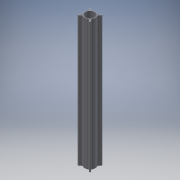
# Autodesk Inventor part: X95_1000mm
Saved by Autodesk Inventor 2016 (Build 200138000, 138)
## iProperties
Created: 2012-04-18
Part Number: X95_1000mm
Document SubType Name: Modeling
Designer: Fabian
Density: 1 g/cm^3
Material: Generic
Appearance: Default
Author: Fabian
Autodesk Inventor part; units mm, degrees
ref_plane "YZ Plane" through (0, 0, 0) normal (1, 0, 0) x (0, 1, 0)
ref_plane "XZ Plane" through (0, 0, 0) normal (0, 1, 0) x (-1, 0, 0)
ref_plane "XY Plane" through (0, 0, 0) normal (0, 0, 1) x (1, 0, 0)
sketch "Sketch1" plane through (0, 0, 0) normal (0, 0, 1) x (1, 0, 0)
  arc A0 (11.6951, -1.7956) -> (0, 0) centre (4.624, -8.8667) ccw
  line L0 (11.6951, -1.7956) -> (21.2005, -11.301)
  arc A1 (21.2005, -11.301) -> (22.9683, -12.0332) centre (22.9683, -9.5332) ccw
  line L1 (22.9683, -12.0332) -> (26.5038, -12.0332)
  arc A2 (26.5038, -12.0332) -> (29.0038, -9.5332) centre (26.5038, -9.5332) ccw
  line L2 (29.0038, -9.5332) -> (29.0038, -5.9977)
  arc A3 (29.0038, -5.9977) -> (28.2716, -4.2299) centre (26.5038, -5.9977) ccw
  line L3 (28.2716, -4.2299) -> (18.7662, 5.2754)
  arc A4 (16.9706, 16.9706) -> (18.7662, 5.2754) centre (25.8373, 12.3465) ccw
  arc A5 (16.9706, 16.9706) -> (16.9706, 53.963) centre (-18.4962, 35.4668) ccw
  arc A6 (18.7662, 65.6581) -> (16.9706, 53.963) centre (25.8373, 58.587) ccw
  line L4 (18.7662, 65.6581) -> (28.2716, 75.1635)
  arc A7 (28.2716, 75.1635) -> (29.0038, 76.9312) centre (26.5038, 76.9312) ccw
  line L5 (29.0038, 76.9312) -> (29.0038, 80.4668)
  arc A8 (29.0038, 80.4668) -> (26.5038, 82.9668) centre (26.5038, 80.4668) ccw
  line L6 (26.5038, 82.9668) -> (22.9683, 82.9668)
  arc A9 (22.9683, 82.9668) -> (21.2005, 82.2345) centre (22.9683, 80.4668) ccw
  line L7 (21.2005, 82.2345) -> (11.6951, 72.7291)
  arc A10 (0, 70.9335) -> (11.6951, 72.7291) centre (4.624, 79.8002) ccw
  arc A11 (0, 70.9335) -> (-36.9924, 70.9335) centre (-18.4962, 35.4668) ccw
  arc A12 (-48.6875, 72.7291) -> (-36.9924, 70.9335) centre (-41.6164, 79.8002) ccw
  line L8 (-48.6875, 72.7291) -> (-58.1929, 82.2345)
  arc A13 (-58.1929, 82.2345) -> (-59.9607, 82.9668) centre (-59.9607, 80.4668) ccw
  line L9 (-59.9607, 82.9668) -> (-63.4962, 82.9668)
  arc A14 (-63.4962, 82.9668) -> (-65.9962, 80.4668) centre (-63.4962, 80.4668) ccw
  line L10 (-65.9962, 80.4668) -> (-65.9962, 76.9312)
  arc A15 (-65.9962, 76.9312) -> (-65.264, 75.1635) centre (-63.4962, 76.9312) ccw
  line L11 (-65.264, 75.1635) -> (-55.7586, 65.6581)
  arc A16 (-53.9629, 53.963) -> (-55.7586, 65.6581) centre (-62.8296, 58.587) ccw
  arc A17 (-53.9629, 53.963) -> (-53.963, 16.9706) centre (-18.4962, 35.4668) ccw
  arc A18 (-55.7586, 5.2754) -> (-53.963, 16.9706) centre (-62.8296, 12.3465) ccw
  line L12 (-55.7586, 5.2754) -> (-65.264, -4.2299)
  arc A19 (-65.264, -4.2299) -> (-65.9962, -5.9977) centre (-63.4962, -5.9977) ccw
  line L13 (-65.9962, -5.9977) -> (-65.9962, -9.5332)
  arc A20 (-65.9962, -9.5332) -> (-63.4962, -12.0332) centre (-63.4962, -9.5332) ccw
  line L14 (-63.4962, -12.0332) -> (-59.9607, -12.0332)
  arc A21 (-59.9607, -12.0332) -> (-58.1929, -11.301) centre (-59.9607, -9.5332) ccw
  line L15 (-58.1929, -11.301) -> (-48.6875, -1.7956)
  arc A22 (-36.9924, 0) -> (-48.6875, -1.7956) centre (-41.6164, -8.8667) ccw
  arc A23 (-36.9924, 0) -> (-18.9962, -4.5301) centre (-18.4962, 35.4668) ccw
  arc A24 (-18.9962, -4.5301) -> (-17.9962, -4.5301) centre (-18.4962, -4.5332) ccw
  arc A25 (-17.9962, -4.5301) -> (0, 0) centre (-18.4962, 35.4668) ccw
  circle A26 centre (-49.9962, 3.9668) radius 3
  circle A27 centre (-49.9962, 66.9668) radius 3
  circle A28 centre (13.0038, 3.9668) radius 3
  circle A29 centre (13.0038, 66.9668) radius 3
  circle A30 centre (-18.4962, 35.4668) radius 36
extrude "Extrusion1" add sketch "Sketch1" along normal blind 1000
body "Solid1"
